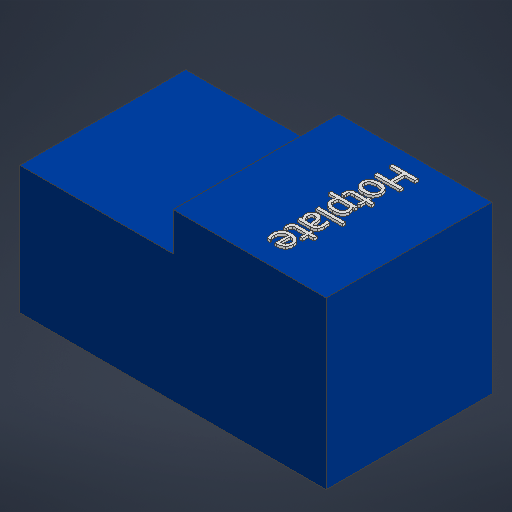
# Autodesk Inventor part: HotPlate
Saved by Autodesk Inventor 2025.1 (Build 291241000, 241)
## iProperties
Created: 2024-10-04
Part Number: HotPlate
Material: Generic
Document SubType Name: Modeling
Designer: jerem
Density: 1 g/cm^3
Appearance: Default
Author: jerem
Autodesk Inventor part; units mm, degrees
ref_plane "YZ Plane" through (0, 0, 0) normal (1, 0, 0) x (0, 1, 0)
ref_plane "XZ Plane" through (0, 0, 0) normal (0, 1, 0) x (-1, 0, 0)
ref_plane "XY Plane" through (0, 0, 0) normal (0, 0, 1) x (1, 0, 0)
sketch "Sketch1" plane through (0, 0, 0) normal (0, 1, 0) x (-1, 0, 0)
  line L0 (-120, -65) -> (120, -65)
  line L1 (120, -65) -> (120, 65)
  line L2 (120, 65) -> (-120, 65)
  line L3 (-120, 65) -> (-120, -65)
  line L4 (-120, -65) -> (120, 65) construction
  line L5 (120, -65) -> (-120, 65) construction
  line L6 (0, 65) -> (0, -65)
  point P0 (0, 0)
  dimension "d0" = 240
  dimension "d1" = 130
  dimension "d4" = 120
  constraints: 14 end point, 4 midpoint, 2 parallel, 2 perpendicular, 1 horizontal
  measures "d0" distance of L2.end L1.end
  measures "d1" distance of L1.end L0.end
  measures "d4" distance between parallel lines of L6 L3
extrude "Extrusion1" add sketch "Sketch1" along normal blind 100
extrude "Extrusion2" add sketch "Sketch1" along normal blind 30 from surface at 100 contours L3 L2 L6 L0
sketch "Sketch2" plane through (0, 130, -65) normal (0, 1, 0) x (1, 0, 0)
  line L0 (78.0568, -13.002) -> (78.0568, -29.4688) construction
  line L1 (78.0568, -29.4688) -> (67.7002, -29.4688) construction
  line L2 (67.7002, -29.4688) -> (67.7002, -13.002) construction
  line L3 (67.7002, -13.002) -> (78.0568, -13.002) construction
  line L4 (57.1654, -29.5498) -> (57.1654, -26.8918)
  line L5 (57.1654, -26.8918) -> (66.9547, -26.8918)
  line L6 (66.9547, -26.8918) -> (66.9547, -17.6859)
  line L7 (66.9547, -17.6859) -> (57.1654, -17.6859)
  line L8 (57.1654, -17.6859) -> (57.1654, -15.0279)
  line L9 (57.1654, -15.0279) -> (77.1654, -15.0279)
  line L10 (77.1654, -15.0279) -> (77.1654, -17.6859)
  line L11 (77.1654, -17.6859) -> (69.321, -17.6859)
  line L12 (69.321, -17.6859) -> (69.321, -26.8918)
  line L13 (69.321, -26.8918) -> (77.1654, -26.8918)
  line L14 (77.1654, -26.8918) -> (77.1654, -29.5498)
  line L15 (77.1654, -29.5498) -> (57.1654, -29.5498)
  spline S0 degree 2 poles (64.6695, -45.7411) (60.8769, -45.7411) (56.744, -42.0944) (56.744, -39.0474) knots 0 0 0 1 2 2 2
  spline S1 degree 2 poles (56.744, -39.0474) (56.744, -35.9193) (61.0066, -32.3375) (64.6695, -32.3375) knots 0 0 0 1 2 2 2
  spline S2 degree 2 poles (64.6695, -32.3375) (68.4296, -32.3375) (72.5949, -36.0328) (72.5949, -39.0474) knots 0 0 0 1 2 2 2
  spline S3 degree 2 poles (72.5949, -39.0474) (72.5949, -42.0944) (68.4458, -45.7411) (64.6695, -45.7411) knots 0 0 0 1 2 2 2
  spline S4 degree 2 poles (64.6695, -43.1317) (67.5868, -43.1317) (70.4231, -41.0085) (70.4231, -39.0474) knots 0 0 0 1 2 2 2
  spline S5 degree 2 poles (70.4231, -39.0474) (70.4231, -37.0863) (67.5868, -34.9469) (64.6695, -34.9469) knots 0 0 0 1 2 2 2
  spline S6 degree 2 poles (64.6695, -34.9469) (61.8331, -34.9469) (58.9158, -37.0863) (58.9158, -39.0474) knots 0 0 0 1 2 2 2
  spline S7 degree 2 poles (58.9158, -39.0474) (58.9158, -40.9923) (61.7845, -43.1317) (64.6695, -43.1317) knots 0 0 0 1 2 2 2
  spline S8 degree 2 poles (56.8737, -52.8723) (56.8737, -50.814) (59.2237, -48.4963) (61.7683, -48.4963) knots 0 0 0 1 2 2 2
  line L16 (61.7683, -48.4963) -> (70.0827, -48.4963)
  line L17 (70.0827, -48.4963) -> (70.0827, -46.7945)
  line L18 (70.0827, -46.7945) -> (72.1735, -46.7945)
  line L19 (72.1735, -46.7945) -> (72.1735, -48.4963)
  line L20 (72.1735, -48.4963) -> (76.4847, -48.4963)
  line L21 (76.4847, -48.4963) -> (76.4847, -51.0247)
  line L22 (76.4847, -51.0247) -> (72.1735, -51.0247)
  line L23 (72.1735, -51.0247) -> (72.1735, -55.6762)
  line L24 (72.1735, -55.6762) -> (70.0827, -55.6762)
  line L25 (70.0827, -55.6762) -> (70.0827, -51.0247)
  line L26 (70.0827, -51.0247) -> (62.9353, -51.0247)
  spline S9 degree 2 poles (62.9353, -51.0247) (61.8007, -51.0247) (60.5528, -51.1057) (60.0179, -51.3812) knots 0 0 0 1 2 2 2
  spline S10 degree 2 poles (60.0179, -51.3812) (59.5479, -51.6082) (59.0779, -52.6292) (59.0779, -53.5044) knots 0 0 0 1 2 2 2
  spline S11 degree 2 poles (59.0779, -53.5044) (59.0779, -54.1203) (59.4506, -55.271) (59.5641, -55.5304) knots 0 0 0 1 2 2 2
  line L27 (59.5641, -55.5304) -> (59.5641, -55.6762)
  line L28 (59.5641, -55.6762) -> (57.2951, -55.6762)
  spline S12 degree 2 poles (57.2951, -55.6762) (57.1006, -54.9631) (56.8737, -53.5044) (56.8737, -52.8723) knots 0 0 0 1 2 2 2
  spline S13 degree 2 poles (65.0746, -70.1171) (61.3145, -70.1171) (56.8737, -66.5352) (56.8737, -63.7962) knots 0 0 0 1 2 2 2
  spline S14 degree 2 poles (56.8737, -63.7962) (56.8737, -62.6778) (57.3923, -60.9599) (57.9271, -60.0684) knots 0 0 0 1 2 2 2
  line L29 (57.9271, -60.0684) -> (51.6387, -60.0684)
  line L30 (51.6387, -60.0684) -> (51.6387, -57.5401)
  line L31 (51.6387, -57.5401) -> (72.1735, -57.5401)
  line L32 (72.1735, -57.5401) -> (72.1735, -60.0684)
  line L33 (72.1735, -60.0684) -> (70.6014, -60.0684)
  spline S15 degree 2 poles (70.6014, -60.0684) (71.4604, -61.0085) (72.5949, -63.3099) (72.5949, -64.6552) knots 0 0 0 1 2 2 2
  spline S16 degree 2 poles (72.5949, -64.6552) (72.5949, -67.2321) (68.5106, -70.1171) (65.0746, -70.1171) knots 0 0 0 1 2 2 2
  spline S17 degree 2 poles (64.7829, -67.5077) (67.3599, -67.5077) (70.1962, -65.8707) (70.1962, -64.0393) knots 0 0 0 1 2 2 2
  spline S18 degree 2 poles (70.1962, -64.0393) (70.1962, -62.9696) (69.24, -60.9599) (68.4944, -60.0684) knots 0 0 0 1 2 2 2
  line L34 (68.4944, -60.0684) -> (59.9693, -60.0684)
  spline S19 degree 2 poles (59.9693, -60.0684) (59.4993, -61.0571) (59.1427, -62.4671) (59.1427, -63.3748) knots 0 0 0 1 2 2 2
  spline S20 degree 2 poles (59.1427, -63.3748) (59.1427, -65.3359) (62.0276, -67.5077) (64.7829, -67.5077) knots 0 0 0 1 2 2 2
  line L35 (57.1654, -75.3197) -> (57.1654, -72.7913)
  line L36 (57.1654, -72.7913) -> (78.0568, -72.7913)
  line L37 (78.0568, -72.7913) -> (78.0568, -75.3197)
  line L38 (78.0568, -75.3197) -> (57.1654, -75.3197)
  spline S21 degree 2 poles (58.7537, -87.3942) (58.5268, -87.0863) (57.7165, -86.049) (57.4733, -85.5628) knots 0 0 0 1 2 2 2
  spline S22 degree 2 poles (57.4733, -85.5628) (57.1168, -84.8983) (56.744, -83.6503) (56.744, -82.5158) knots 0 0 0 1 2 2 2
  spline S23 degree 2 poles (56.744, -82.5158) (56.744, -81.5919) (57.4409, -79.9226) (58.073, -79.2905) knots 0 0 0 1 2 2 2
  spline S24 degree 2 poles (58.073, -79.2905) (58.6889, -78.6908) (60.5041, -77.9615) (61.509, -77.9615) knots 0 0 0 1 2 2 2
  spline S25 degree 2 poles (61.509, -77.9615) (63.0649, -77.9615) (65.2691, -79.2743) (65.9012, -80.7005) knots 0 0 0 1 2 2 2
  spline S26 degree 2 poles (65.9012, -80.7005) (66.4847, -81.9647) (66.9223, -85.4007) (67.0357, -87.3942) knots 0 0 0 1 2 2 2
  line L39 (67.0357, -87.3942) -> (67.522, -87.3942)
  spline S27 degree 2 poles (67.522, -87.3942) (68.3972, -87.3942) (69.4831, -86.8594) (69.791, -86.3731) knots 0 0 0 1 2 2 2
  spline S28 degree 2 poles (69.791, -86.3731) (70.0989, -85.8869) (70.2934, -84.4931) (70.2934, -83.7475) knots 0 0 0 1 2 2 2
  spline S29 degree 2 poles (70.2934, -83.7475) (70.2934, -82.8723) (69.7748, -80.506) (69.2724, -79.3229) knots 0 0 0 1 2 2 2
  line L40 (69.2724, -79.3229) -> (69.2724, -79.177)
  line L41 (69.2724, -79.177) -> (71.8494, -79.177)
  spline S30 degree 2 poles (71.8494, -79.177) (72.0438, -79.874) (72.5301, -82.4834) (72.5301, -83.7637) knots 0 0 0 1 2 2 2
  spline S31 degree 2 poles (72.5301, -83.7637) (72.5301, -85.3197) (72.0438, -87.4428) (71.4118, -88.2856) knots 0 0 0 1 2 2 2
  spline S32 degree 2 poles (71.4118, -88.2856) (70.7959, -89.1122) (68.8348, -89.9226) (67.4247, -89.9226) knots 0 0 0 1 2 2 2
  line L42 (67.4247, -89.9226) -> (57.1654, -89.9226)
  line L43 (57.1654, -89.9226) -> (57.1654, -87.3942)
  line L44 (57.1654, -87.3942) -> (58.7537, -87.3942)
  line L45 (60.8607, -87.3942) -> (65.026, -87.3942)
  spline S33 degree 2 poles (65.026, -87.3942) (64.945, -86.4866) (64.6695, -83.7475) (64.4101, -82.8885) knots 0 0 0 1 2 2 2
  spline S34 degree 2 poles (64.4101, -82.8885) (64.1022, -81.8837) (62.8218, -80.5709) (61.6873, -80.5709) knots 0 0 0 1 2 2 2
  spline S35 degree 2 poles (61.6873, -80.5709) (60.3907, -80.5709) (59.0779, -82.0295) (59.0779, -83.4234) knots 0 0 0 1 2 2 2
  spline S36 degree 2 poles (59.0779, -83.4234) (59.0779, -84.6065) (60.0989, -86.5514) (60.8607, -87.3942) knots 0 0 0 1 2 2 2
  spline S37 degree 2 poles (56.8737, -98.0101) (56.8737, -95.9517) (59.2237, -93.6341) (61.7683, -93.6341) knots 0 0 0 1 2 2 2
  line L46 (61.7683, -93.6341) -> (70.0827, -93.6341)
  line L47 (70.0827, -93.6341) -> (70.0827, -91.9323)
  line L48 (70.0827, -91.9323) -> (72.1735, -91.9323)
  line L49 (72.1735, -91.9323) -> (72.1735, -93.6341)
  line L50 (72.1735, -93.6341) -> (76.4847, -93.6341)
  line L51 (76.4847, -93.6341) -> (76.4847, -96.1624)
  line L52 (76.4847, -96.1624) -> (72.1735, -96.1624)
  line L53 (72.1735, -96.1624) -> (72.1735, -100.814)
  line L54 (72.1735, -100.814) -> (70.0827, -100.814)
  line L55 (70.0827, -100.814) -> (70.0827, -96.1624)
  line L56 (70.0827, -96.1624) -> (62.9353, -96.1624)
  spline S38 degree 2 poles (62.9353, -96.1624) (61.8007, -96.1624) (60.5528, -96.2435) (60.0179, -96.519) knots 0 0 0 1 2 2 2
  spline S39 degree 2 poles (60.0179, -96.519) (59.5479, -96.7459) (59.0779, -97.767) (59.0779, -98.6422) knots 0 0 0 1 2 2 2
  spline S40 degree 2 poles (59.0779, -98.6422) (59.0779, -99.2581) (59.4506, -100.4088) (59.5641, -100.6681) knots 0 0 0 1 2 2 2
  line L57 (59.5641, -100.6681) -> (59.5641, -100.814)
  line L58 (59.5641, -100.814) -> (57.2951, -100.814)
  spline S41 degree 2 poles (57.2951, -100.814) (57.1006, -100.1009) (56.8737, -98.6422) (56.8737, -98.0101) knots 0 0 0 1 2 2 2
  spline S42 degree 2 poles (56.825, -109.1932) (56.825, -105.5952) (60.8607, -101.6406) (64.5884, -101.6406) knots 0 0 0 1 2 2 2
  spline S43 degree 2 poles (64.5884, -101.6406) (68.2513, -101.6406) (72.5949, -105.4817) (72.5949, -108.5774) knots 0 0 0 1 2 2 2
  spline S44 degree 2 poles (72.5949, -108.5774) (72.5949, -109.9712) (71.7845, -112.1268) (70.9255, -112.921) knots 0 0 0 1 2 2 2
  spline S45 degree 2 poles (70.9255, -112.921) (70.0665, -113.7313) (67.5868, -114.5903) (65.7878, -114.5903) knots 0 0 0 1 2 2 2
  line L59 (65.7878, -114.5903) -> (64.4101, -114.5903)
  line L60 (64.4101, -114.5903) -> (64.4101, -104.2013)
  spline S46 degree 2 poles (64.4101, -104.2013) (61.8007, -104.2013) (59.0293, -106.827) (59.0293, -109.1608) knots 0 0 0 1 2 2 2
  spline S47 degree 2 poles (59.0293, -109.1608) (59.0293, -109.9874) (59.402, -111.5919) (59.6938, -112.2402) knots 0 0 0 1 2 2 2
  spline S48 degree 2 poles (59.6938, -112.2402) (60.0179, -112.921) (60.5852, -113.861) (60.8445, -114.1689) knots 0 0 0 1 2 2 2
  line L61 (60.8445, -114.1689) -> (60.8445, -114.3148)
  line L62 (60.8445, -114.3148) -> (58.0892, -114.3148)
  spline S49 degree 2 poles (58.0892, -114.3148) (57.9109, -113.8772) (57.3923, -112.5482) (57.2464, -112.0295) knots 0 0 0 1 2 2 2
  spline S50 degree 2 poles (57.2464, -112.0295) (57.0357, -111.3002) (56.825, -110.1009) (56.825, -109.1932) knots 0 0 0 1 2 2 2
  spline S51 degree 2 poles (66.3388, -112.1268) (67.3599, -112.0944) (68.851, -111.673) (69.3534, -111.2678) knots 0 0 0 1 2 2 2
  spline S52 degree 2 poles (69.3534, -111.2678) (69.9207, -110.8302) (70.5203, -109.4526) (70.5203, -108.4315) knots 0 0 0 1 2 2 2
  spline S53 degree 2 poles (70.5203, -108.4315) (70.5203, -107.4266) (69.9207, -106.0166) (69.3372, -105.4331) knots 0 0 0 1 2 2 2
  spline S54 degree 2 poles (69.3372, -105.4331) (68.7375, -104.8658) (67.2951, -104.2824) (66.3388, -104.2013) knots 0 0 0 1 2 2 2
  line L63 (66.3388, -104.2013) -> (66.3388, -112.1268)
  point P0 (0, -65)
  point P1 (67.1766, -110.0367)
  constraints: 2 other
extrude "Extrusion3" add sketch "Sketch2" along normal blind 2
body "Solid1"
